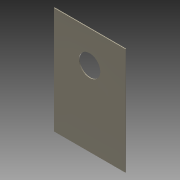
# Autodesk Inventor part: TO220 Thermal Film
Saved by Autodesk Inventor 2015 (Build 190159000, 159)
## iProperties
Created: 2016-01-19
Part Number: TO220 Thermal Film
Material: Generic
Document SubType Name: Modeling
Designer: Kyle
Density: 1 g/cm^3
Appearance: Light Beige
Author: Kyle
Autodesk Inventor part; units mm, degrees
ref_plane "YZ Plane" through (0, 0, 0) normal (1, 0, 0) x (0, 1, 0)
ref_plane "XZ Plane" through (0, 0, 0) normal (0, 1, 0) x (-1, 0, 0)
ref_plane "XY Plane" through (0, 0, 0) normal (0, 0, 1) x (1, 0, 0)
sketch "Sketch1" plane through (0, 0, 0) normal (0, 0, 1) x (1, 0, 0)
  line L0 (0, 0) -> (12.7, 0)
  line L1 (12.7, 0) -> (12.7, 19.05)
  line L2 (12.7, 19.05) -> (0, 19.05)
  line L3 (0, 19.05) -> (0, 0)
  dimension "d0" = 19.05
  dimension "d1" = 12.7
  constraints: 8 end point, 2 parallel, 1 horizontal, 1 perpendicular
  measures "d0" distance of L0.end L1.end
  measures "d1" distance of L0.start L0.end
extrude "Extrusion1" add sketch "Sketch1" along normal blind 0.1397
sketch "Sketch2" plane through (0, 0, 0.1397) normal (0, 0, 1) x (1, 0, 0)
  circle A0 centre (6.35, 13.3299) radius 1.905
  line L0 (12.7, 0) -> (12.7, 19.05) projected
  line L1 (12.7, 19.05) -> (0, 19.05) projected
  point P0 (0, 0)
  dimension "d4" = 6.35
  dimension "d5" = 5.7201
  dimension "d6" = 3.81
  constraints: 1 centre point
  measures "d4" distance from line of L0 A0.centre
  measures "d5" distance from line of A0.centre L1
  measures "d6" diameter of A0
extrude "Extrusion2" cut sketch "Sketch2" against normal blind 0.1397
body "Solid1"
